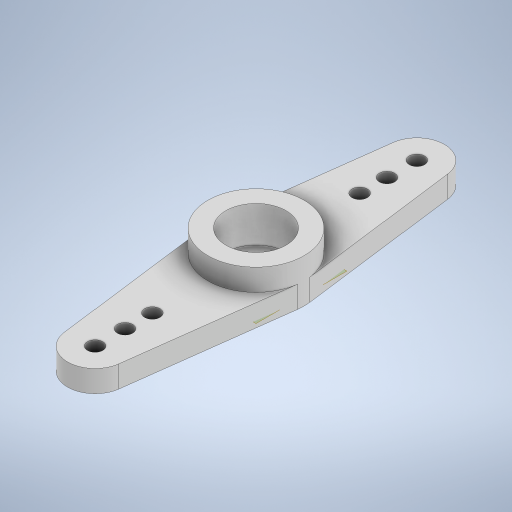
# Autodesk Inventor part: Standard Servo Horn - White Propellor
Saved by Autodesk Inventor 2023 (Build 270158000, 158)
## iProperties
Created: 2023-09-05
Part Number: Standard Servo Horn - White Propellor
Material: Generic
Document SubType Name: Modeling
Designer: Nate
Density: 1 g/cm^3
Appearance: Default
Author: Nate
Autodesk Inventor part; units mm, degrees
ref_plane "YZ Plane" through (0, 0, 0) normal (1, 0, 0) x (0, 1, 0)
ref_plane "XZ Plane" through (0, 0, 0) normal (0, 1, 0) x (-1, 0, 0)
ref_plane "XY Plane" through (0, 0, 0) normal (0, 0, 1) x (1, 0, 0)
sketch "Sketch1" plane through (0, 0, 0) normal (0, 1, 0) x (-1, 0, 0)
  circle A0 centre (0, 0) radius 1.375
  circle A1 centre (0, 0) radius 2.75
  circle A2 centre (0, 0) radius 3.785
  circle A3 centre (0, 0) radius 4.4
  circle A4 centre (-0.0015, -14.74) radius 2.52
  circle A5 centre (-0.0015, -14.74) radius 0.7
  circle A6 centre (0, -12) radius 0.7
  circle A7 centre (0, -9.5) radius 0.7
  line L0 (4.364, -0.5616) -> (2.4979, -15.0617)
  line L1 (-4.3641, -0.5608) -> (-2.5009, -15.0612)
  line L2 (-4.364, 0.5616) -> (-2.4979, 15.0617)
  line L3 (4.3641, 0.5608) -> (2.5009, 15.0612)
  circle A8 centre (0, 9.5) radius 0.7
  circle A9 centre (0, 12) radius 0.7
  circle A10 centre (0.0015, 14.74) radius 2.52
  circle A11 centre (0.0015, 14.74) radius 0.7
  dimension "d0" = 2.75
  dimension "d1" = 5.5
  dimension "d2" = 7.57
  dimension "d3" = 8.8
  dimension "d4" = 5.04
  dimension "d5" = 14.74
  dimension "d6" = 1.4
  dimension "d7" = 1.4
  dimension "d8" = 1.4
  dimension "d9" = 9.5
  dimension "d10" = 12
  dimension "d13" = 360
  constraints: 12 centre point, 8 end point, 6 coincident, 6 point on circle, 4 tangent, 29 other
  measures "d0" diameter of A0
  measures "d1" diameter of A1
  measures "d2" diameter of A2
  measures "d3" diameter of A3
  measures "d4" diameter of A4
  measures "d5" distance of A4.centre point (0, 0)
  measures "d6" diameter of A5
  measures "d7" diameter of A6
  measures "d8" diameter of A7
  measures "d9" distance of A7.centre point (0, 0)
  measures "d10" distance of A6.centre point (0, 0)
extrude "Extrusion1" add sketch "Sketch1" along normal blind 2 contours A3 L2 A10 A9 L3 | L0 A4 A6 L1 A3 | A10 A9 | A4 A6 picked at (-0.632, 13.1055) picked at (-0.6336, -13.105)
extrude "Extrusion2" add sketch "Sketch1" along normal blind 4 contours A3
extrude "Extrusion3" add sketch "Sketch1" along normal blind 4 and the other way blind 0.45 contours A2
ref_plane "Work Plane1" through (0, 0.58, 0) normal (0, -1, 0) x (1, 0, 0)
sketch "Sketch2" plane through (0, 0.58, 0) normal (0, -1, 0) x (1, 0, 0)
  circle A0 centre (0, 0) radius 2.75
  circle A1 centre (0, 0) radius 1.375
  dimension "d26" = 5.5
  dimension "d27" = 2.75
  constraints: 2 centre point, 2 coincident
  measures "d26" diameter of A0
  measures "d27" diameter of A1
extrude "Extrusion5" add sketch "Sketch2" against normal blind 0.12
body "Solid1"
